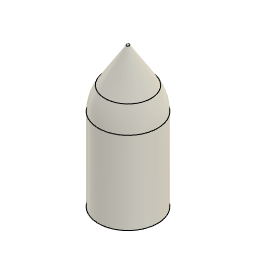
Razzetto v2 (Autodesk Fusion 360 design; units mm, degrees)
Autodesk Fusion 360 part; units mm, degrees
sketch "Schizzo2" plane through (0, 0, 0) normal (0, 1, 0) x (1, 0, 0)
  line L0 (4.25, 0) -> (6.25, 0)
  line L1 (6.25, 0) -> (6.25, -17.4188)
  line L2 (6.25, 0) -> (6.25, -20)
  line L3 (0.2968, -29.5251) -> (4.882, -22.1888)
  line L4 (6.25, 0) -> (4.25, 0)
  line L5 (4.25, -5.8409) -> (4.25, -17.4188)
  line L6 (0.5, -20) -> (0.5, -23)
  line L7 (0, -23) -> (0, -29.6896)
  line L8 (0.5, -20) -> (0.5, -0.866)
  arc A0 (0.5, -0.866) -> (0, 1) centre (0, 0) ccw
  line L9 (0, 1) -> (0, -23)
  line L10 (4.25, 0) -> (2.25, 0)
  line L11 (2.25, 0) -> (12.25, 0) construction
  line L12 (2.25, 0) -> (3.5942, -2.8825)
  arc A1 (4.25, -5.8409) -> (3.5942, -2.8825) centre (-2.75, -5.8409) ccw
  arc A2 (4.882, -22.1888) -> (6.25, -17.4188) centre (-2.75, -17.4188) ccw
  line L13 (0.9375, -28.5) -> (0, -28.5) construction
  arc A3 (0, -29.6896) -> (0.2968, -29.5251) centre (0, -29.3396) ccw
  line L14 (2.0165, -23) -> (3.186, -21.1288)
  arc A4 (3.186, -21.1288) -> (4.25, -17.4188) centre (-2.75, -17.4188) ccw
  line L15 (4.25, -5.8409) -> (4.25, -17.4188)
  line L16 (0.5, -23) -> (2.0165, -23)
  line L17 (0.5, -23) -> (0.5, -26)
  line L18 (0.5, -26) -> (0, -26)
  dimension "d9" = 6.25
  dimension "d13" = 20
  dimension "d15" = 2
  dimension "d17" = 3
  dimension "d18" = 2
  dimension "d20" = 2
  dimension "d21" = 65
  dimension "d23" = 7
  dimension "d24" = 9
  dimension "d25" = 0.35
  dimension "d28" = 3
  constraint horizontal L0
  constraint perpendicular L0 L1
  constraint perpendicular L0 L2
  constraint perpendicular L1 L4
  constraint perpendicular L0 L5
  constraint coincident A0.centre origin
  constraint perpendicular L5 L10
  constraint horizontal L11
  constraint tangent L5 A1
  constraint tangent L12 A1
  constraint coincident L2.end L3
  constraint tangent L3 A2
  constraint tangent L1 A2
  constraint horizontal L13
  constraint coincident L3 L13.start
  constraint coincident L7 L13.end
  constraint tangent L3 A3
  constraint concentric A2 A4
  constraint tangent L14 A4
  constraint tangent A4 L15
  constraint perpendicular L6 L16
  constraint perpendicular L16 L17
  constraint coincident L7 L18.end
  constraint perpendicular L7 L18
  measures "d9" distance of A0.centre L0.end
  measures "d13" distance of L0.end L2.end
  measures "d15" distance of L0.end L0.start
  measures "d17" distance of L6.start L6.end
  measures "d18" diameter of A0
  measures "d20" distance of L0.start L10.end
  measures "d21" angle of L11 L12
  measures "d23" radius of A1
  measures "d24" radius of A2
  measures "d25" radius of A3
  measures "d28" distance of L6.end L17.end
revolve "Rivoluzione3" add sketch "Schizzo2" angle 360 about axis through (0, 0, -1) along (0, 0, 1) contours L0 L1 L2 L3 L4 L5 L7 L10 L12 A1 A2 A3 L14 A4 L15 L16 L17 L18 makes body 1
ref_plane "Piano di lavoro1" through (0, -3, 0) normal (0, 1, 0) x (0, 0, 1)
revolve "Rivoluzione4" add sketch "Schizzo2" angle 360 about axis through (0, 0, -1) along (0, 0, 1) separate body contours L6 L7 L8 A0 L9 L17 L18 makes body 2
revolve "Rivoluzione2" [rolled back] along angle 360
sketch "Schizzo3" plane through (0, 0, 0) normal (0, 1, 0) x (1, 0, 0)
  line L0 (0, 1) -> (0, -23)
  constraint vertical L0
revolve "Rivoluzione1" [rolled back] along angle 360
equation "d9 = ( 12.5 / 2 ) * 1 mm"
named bodies: "razzo", "fiammifero"
